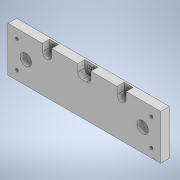
# Autodesk Inventor part: cpc_module_weight_tool_1x2_v2
Saved by Autodesk Inventor 2021 (Build 250183000, 183)
## iProperties
Created: 2020-09-18
Part Number: cpc_module_weight_tool_1x2_v2
Material: Generic
Document SubType Name: Modeling
Designer: jones105
Density: 1 g/cm^3
Appearance: Default
Author: jones105
Autodesk Inventor part; units mm, degrees
ref_plane "YZ Plane" through (0, 0, 0) normal (1, 0, 0) x (0, 1, 0)
ref_plane "XZ Plane" through (0, 0, 0) normal (0, 1, 0) x (-1, 0, 0)
ref_plane "XY Plane" through (0, 0, 0) normal (0, 0, 1) x (1, 0, 0)
sketch "Sketch1" plane through (0, 0, 0) normal (0, 0, 1) x (1, 0, 0)
  line L0 (0, 0) -> (85, 0)
  line L1 (85, 0) -> (85, 25)
  line L2 (85, 25) -> (0, 25)
  line L3 (0, 25) -> (0, 0)
  dimension "d0" = 85
  dimension "d1" = 25
  constraints: 8 end point, 2 parallel, 1 horizontal, 1 perpendicular
  measures "d0" distance between parallel lines of L1 L3
  measures "d1" distance between parallel lines of L0 L2
extrude "Extrusion1" add sketch "Sketch1" along normal blind 6.35
sketch "Sketch2" plane through (0, 0, 0) normal (0, 0, -1) x (-1, 0, 0)
  line L0 (11.8425, 12.5) -> (-122.9344, 12.5) construction
  line L1 (-85, 25) -> (0, 25) construction
  line L2 (0, 0) -> (-85, 0) construction
  line L3 (0, 25) -> (0, 0) construction
  line L4 (-85, 0) -> (-85, 25) construction
  point P0 (-10, 12.5)
  point P1 (-75, 12.5)
  dimension "d4" = 25
  dimension "d5" = 12.5
  dimension "d6" = 65
  dimension "d7" = 10
  dimension "d8" = 85
  constraints: 2 end point, 2 point on line, 1 horizontal
  measures "d4" distance between parallel lines of L1 L2
  measures "d5" distance between parallel lines of L2 L0
  measures "d6" distance of point (-75, 12.5) point (-10, 12.5)
  measures "d7" distance from line of L3 point (-10, 12.5)
  measures "d8" distance between parallel lines of L4 L3
hole "Hole1" at (10, 12.5, 0) at (75, 12.5, 0) direction (0, 0, 1) diameter 6.35 end through all
sketch "Sketch3" plane through (0, 0, 0) normal (0, 0, -1) x (-1, 0, 0)
  line L0 (0, 0) -> (-85, 0) projected
  line L1 (-85, 25) -> (0, 25) projected
  line L2 (0, 0) -> (-85, 0)
  line L3 (-85, 0) -> (-85, 25)
  line L4 (-85, 25) -> (0, 25)
  line L5 (0, 25) -> (0, 0)
  circle A0 centre (-10, 12.5) radius 3.175 projected
  circle A1 centre (-10, 12.5) radius 5
  circle A2 centre (-75, 12.5) radius 3.175 projected
  circle A3 centre (-75, 12.5) radius 5
  line L6 (-20, 4) -> (-65, 4)
  line L7 (-65, 4) -> (-65, 21)
  line L8 (-65, 21) -> (-20, 21)
  line L9 (-20, 21) -> (-20, 4)
  line L10 (-23, 17) -> (-62, 17)
  line L11 (-62, 19) -> (-23, 19)
  arc A4 (-23, 17) -> (-23, 19) centre (-23, 18) ccw
  arc A5 (-62, 19) -> (-62, 17) centre (-62, 18) ccw
  dimension "d16" = 10
  dimension "d17" = 10
  dimension "d18" = 45
  dimension "d19" = 85
  dimension "d20" = 20
  dimension "d21" = 5
  dimension "d22" = 17
  dimension "d23" = 25
  dimension "d24" = 4
  dimension "d25" = 2
  dimension "d26" = 2
  dimension "d27" = 3
  dimension "d28" = 3
  constraints: 20 end point, 5 parallel, 4 centre point, 4 point on circle, 4 tangent, 3 horizontal, 2 coincident, 2 perpendicular
  measures "d16" diameter of A1
  measures "d17" diameter of A3
  measures "d18" distance between parallel lines of L7 L9
  measures "d19" distance between parallel lines of L3 L5
  measures "d20" distance between parallel lines of L5 L9
  measures "d21" distance edge to line of A1 L9
  measures "d22" distance between parallel lines of L8 L6
  measures "d23" distance between parallel lines of L0 L1
  measures "d24" distance between parallel lines of L1 L8
  measures "d25" distance between parallel lines of L10 L11
  measures "d26" distance between parallel lines of L8 L11
  measures "d27" distance from line of L9 A4.centre
  measures "d28" distance from line of L7 A5.centre
extrude "Extrusion2" cut sketch "Sketch3" against normal blind 1.5 contours L0 L3 L1 L5 | L10 A5 L11 A4
chamfer "Chamfer1" distance 0.5 angle 45 6 edges at (15, 12.5, 0) (20, 12.5, 0) (42.5, 21, 0) (65, 12.5, 0) (42.5, 4, 0) (80, 12.5, 0)
sketch "Sketch4" plane through (0, 0, 6.35) normal (0, 0, 1) x (1, 0, 0)
  line L0 (91.97, 21.07) -> (-14.1412, 21.07) construction
  circle A0 centre (75, 12.5) radius 3.175 construction
  circle A1 centre (10, 12.5) radius 3.175 construction
  line L1 (63.275, 17.0371) -> (63.275, 27.1253) construction
  line L2 (43.675, 17.4706) -> (43.675, 26.9283) construction
  line L3 (41.425, 17.4706) -> (41.425, 28.8987) construction
  line L4 (21.825, 18.5093) -> (21.825, 30.9592) construction
  line L5 (70.2986, 22.57) -> (18.3832, 22.57) construction
  point P0 (0, 0)
  point P1 (63.275, 21.07)
  point P2 (21.825, 21.07)
  point P3 (43.675, 21.07)
  point P4 (41.425, 21.07)
  point P5 (63.275, 22.57)
  point P6 (43.675, 22.57)
  point P7 (41.425, 22.57)
  point P8 (21.825, 22.57)
  dimension "d34" = 11.725
  dimension "d35" = 8.57
  dimension "d36" = 31.325
  dimension "d37" = 33.575
  dimension "d38" = 53.175
  dimension "d39" = 11.825
  dimension "d56" = 1.5
  constraints: 12 end point, 12 point on line, 4 vertical, 2 horizontal
  measures "d34" horizontal distance of point (63.275, 21.07) A0.centre
  measures "d35" distance from line of L0 A0.centre
  measures "d36" horizontal distance of point (43.675, 21.07) A0.centre
  measures "d37" horizontal distance of point (41.425, 21.07) A0.centre
  measures "d38" horizontal distance of point (21.825, 21.07) A0.centre
  measures "d39" horizontal distance of A1.centre point (21.825, 21.07)
  measures "d56" distance between parallel lines of L0 L5
hole "Hole2" at (63.275, 21.07, 6.35) at (21.825, 21.07, 6.35) at (43.675, 21.07, 6.35) at (41.425, 21.07, 6.35) at (63.275, 22.57, 6.35) at (43.675, 22.57, 6.35) at (41.425, 22.57, 6.35) at (21.825, 22.57, 6.35) direction (0, 0, -1) diameter 1.2 end through all
sketch "Sketch5" plane through (0, 0, 6.35) normal (0, 0, 1) x (1, 0, 0)
  line L0 (85, 25) -> (0, 25) projected
  line L1 (65.775, 25) -> (65.775, 21.07)
  line L2 (60.775, 21.07) -> (60.775, 25)
  arc A0 (60.775, 21.07) -> (65.775, 21.07) centre (63.275, 21.07) ccw
  line L3 (24.325, 25) -> (19.325, 25)
  line L4 (24.325, 21.07) -> (24.325, 25)
  line L5 (19.325, 25) -> (19.325, 21.07)
  line L6 (20, 4) -> (20, 21) projected
  arc A1 (19.325, 21.07) -> (24.325, 21.07) centre (21.825, 21.07) ccw
  circle A2 centre (63.275, 21.07) radius 0.6 projected
  circle A3 centre (21.825, 21.07) radius 0.6 projected
  line L7 (65.775, 25) -> (60.775, 25)
  line L8 (46.175, 25) -> (38.925, 25)
  line L9 (38.925, 25) -> (38.925, 21.07)
  line L10 (38.925, 21.07) -> (46.175, 21.07)
  line L11 (46.175, 21.07) -> (46.175, 25)
  arc A4 (43.675, 18.57) -> (46.175, 21.07) centre (43.675, 21.07) ccw
  arc A5 (38.925, 21.07) -> (41.425, 18.57) centre (41.425, 21.07) ccw
  line L12 (41.425, 18.57) -> (43.675, 18.57)
  circle A6 centre (43.675, 21.07) radius 0.6 projected
  circle A7 centre (41.425, 21.07) radius 0.6 projected
  point P0 (0, 0)
  dimension "d47" = 5
  dimension "d48" = 5
  dimension "d49" = 2.5
  dimension "d50" = 2.5
  constraints: 22 end point, 8 point on circle, 8 tangent, 4 centre point, 4 concentric, 4 parallel, 4 point on line, 1 collinear, 1 horizontal, 1 perpendicular, 1 vertical
  measures "d47" distance between parallel lines of L2 L1
  measures "d48" distance between parallel lines of L5 L4
  measures "d49" distance from line of L11 A4.centre
  measures "d50" distance from line of L9 A5.centre
extrude "Extrusion3" cut sketch "Sketch5" against normal blind 3.85 contours L1 A0 L2 L0 | L11 L10 A6 A7 L9 L0 | A4 L12 A5 L10 A7 A6 | L4 A1 L5 L0
chamfer "Chamfer2" distance 0.5 angle 45 4 edges at (63.275, 21.67, 2.5) (43.675, 21.67, 2.5) (41.425, 21.67, 2.5) (21.825, 21.67, 2.5)
chamfer "Chamfer3" distance 0.5 angle 45 4 edges at (63.275, 23.17, 2.5) (43.675, 23.17, 2.5) (41.425, 23.17, 2.5) (21.825, 23.17, 2.5)
sketch "Sketch6" plane through (0, 0, 6.35) normal (0, 0, 1) x (1, 0, 0)
  line L0 (5, 20) -> (5, 5) construction
  line L1 (5, 5) -> (80, 5) construction
  line L2 (20.5, 4.5) -> (64.5, 4.5) construction
  line L3 (80, 5) -> (80, 20) construction
  line L4 (80, 20) -> (5, 20) construction
  line L5 (0, 25) -> (0, 0) construction
  line L6 (19.325, 25) -> (0, 25) construction
  line L7 (0, 0) -> (85, 0) construction
  line L8 (85, 0) -> (85, 25) construction
  dimension "d60" = 5
  dimension "d61" = 5
  dimension "d62" = 5
  dimension "d63" = 5
  constraints: 8 end point, 4 coincident, 2 perpendicular, 1 parallel, 1 vertical
  measures "d60" distance between parallel lines of L5 L0
  measures "d61" distance between parallel lines of L6 L4
  measures "d62" distance between parallel lines of L7 L1
  measures "d63" distance between parallel lines of L8 L3
hole "Hole3" at (80, 20, 6.35) at (80, 5, 6.35) at (5, 20, 6.35) at (5, 5, 6.35) direction (0, 0, -1) diameter 1.567 depth 6.3 tip angle 118 thread size "M2x0.4" class "6H" standard "ANSI Metric M Profile"
equation "\"d5\" = 0.5 * d4"
equation "\"d7\" = -0.5 * d6 + 0.5 * d8"
equation "\"d17\" = d16"
equation "\"d20\" = -0.5 * d18 + 0.5 * d19"
equation "\"d24\" = -0.5 * d22 + 0.5 * d23"
body "Solid1"
